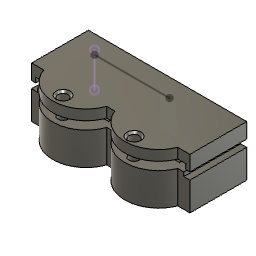
nixie_holder v9 (Autodesk Fusion 360 design; units mm, degrees)
Autodesk Fusion 360 part; units mm, degrees
sketch "Skizze1" plane through (0, 0, 0) normal (0, 1, 0) x (1, 0, 0)
  circle A0 centre (0, 0) radius 7
  circle A1 centre (0, 0) radius 12.5
  line L0 (0, 0) -> (13, 0)
  line L1 (13, 0) -> (13, -2)
  line L2 (13, -2) -> (0, -2)
  line L3 (0, -2) -> (0, 0)
  line L4 (0, 0) -> (-13, 0)
  line L5 (-13, 0) -> (-13, -2)
  line L6 (-13, -2) -> (0, -2)
  line L7 (0, -2) -> (0, 0)
  line L8 (14, -14) -> (-14, -14)
  line L9 (-14, -14) -> (-14, 14)
  line L10 (-14, 14) -> (14, 14)
  line L11 (14, 14) -> (14, -14)
  line L12 (14, -14) -> (-14, 14) construction
  line L13 (-14, -14) -> (14, 14) construction
  line L14 (15.5, 15.5) -> (-15.5, 15.5)
  line L15 (-15.5, 15.5) -> (-15.5, -15.5)
  line L16 (-15.5, -15.5) -> (15.5, -15.5)
  line L17 (15.5, -15.5) -> (15.5, 15.5)
  line L18 (15.5, 15.5) -> (-15.5, -15.5) construction
  line L19 (-15.5, 15.5) -> (15.5, -15.5) construction
  line L20 (-13, -2) -> (-13, -14)
  line L21 (-13, 0) -> (-15.5, 0)
  line L22 (13, -2) -> (14, -2)
  line L23 (13, 0) -> (15.5, 0)
  line L24 (15.5, -2) -> (14, -2)
  line L25 (-13, -2) -> (-15.5, -2)
  line L26 (-15.5, 15.5) -> (15.5, 15.5)
  line L27 (15.5, 15.5) -> (15.5, 14)
  line L28 (15.5, 14) -> (-15.5, 14)
  line L29 (-15.5, 14) -> (-15.5, 15.5)
  dimension "d1" = 14
  dimension "d2" = 25
  dimension "d3" = 28
  dimension "d4" = 31
  dimension "d5" = 31
  constraint coincident A0.centre A1.centre
  constraint horizontal L0
  constraint vertical L1
  constraint horizontal L2
  constraint vertical L3
  constraint horizontal L4
  constraint vertical L5
  constraint horizontal L6
  constraint vertical L7
  constraint perpendicular L8 L9
  constraint parallel L8 L10
  constraint parallel L9 L11
  constraint horizontal L8
  constraint coincident L12 A0.centre
  constraint coincident L13 A0.centre
  constraint perpendicular L14 L15
  constraint parallel L14 L16
  constraint parallel L15 L17
  constraint horizontal L14
  constraint coincident L18 A0.centre
  constraint coincident L19 A0.centre
  constraint perpendicular L6 L20
  constraint midpoint L15 L21.end
  constraint coincident L11 L22.end
  constraint perpendicular L11 L22
  constraint midpoint L17 L23.end
  constraint coincident L17 L24.start
  constraint perpendicular L11 L24
  constraint coincident L15 L25.end
  constraint perpendicular L15 L25
  constraint horizontal L26
  constraint vertical L27
  constraint horizontal L28
  constraint vertical L29
  constraint coincident L17 L27.end
  measures "d1" diameter of A0
  measures "d2" diameter of A1
  measures "d3" distance of L8.end L9.end
  measures "d4" distance of L15.end L16.end
  measures "d5" distance of L14.end L15.end
extrude "Extrusion1" add sketch "Skizze1" along normal blind 12 contours A0 A1 L0 L2 | A0 A1 L0 L4 | A0 A1 L4 L6 | A0 A1 L2 L6 | A1 L0 L1 L2 | A1 L4 L5 L6 | L1 L11 L22 L23 | L5 L9 L21 L25 | L11 L17 L23 L24 | L11 L17 L23 L28 | L9 L15 L21 L28 | L9 L15 L21 L25 | L8 L9 L11 L15 L16 L17 L24 L25 makes body 1
sketch "Skizze2" plane through (0, 12, 0) normal (0, 1, 0) x (-1, 0, 0)
  line L0 (14, 2) -> (12.339, 2)
  arc A0 (12.339, 2) -> (-12.339, 2) centre (0, 0) ccw
  line L1 (-12.339, 2) -> (-14, 2)
  line L2 (-14, 2) -> (-14, 14)
  line L3 (-14, 14) -> (14, 14)
  line L4 (14, 14) -> (14, 2)
  circle A1 centre (0, 0) radius 7
  arc A2 (-12.5, 0) -> (12.5, 0) centre (0, 0) ccw
  line L5 (12.5, 0) -> (14, 0)
  line L6 (14, 0) -> (14, -14)
  line L7 (14, -14) -> (15.5, -14)
  line L8 (15.5, -14) -> (15.5, 15.5)
  line L9 (15.5, 15.5) -> (-15.5, 15.5)
  line L10 (-15.5, 15.5) -> (-15.5, -14)
  line L11 (-15.5, -14) -> (-14, -14)
  line L12 (-14, -14) -> (-14, 0)
  line L13 (-14, 0) -> (-12.5, 0)
  circle A3 centre (0, 0) radius 7
  circle A4 centre (0, 0) radius 8.5
  dimension "d8" = 17
  constraint coincident A0.centre A1.centre
  constraint concentric A3 A4
  measures "d8" diameter of A4
extrude "Extrusion2" cut sketch "Skizze2" against normal blind 15 contours A4 bodies 1
sketch "Skizze3" plane through (0, 12, 0) normal (0, 1, 0) x (-1, 0, 0)
  circle A0 centre (0, 0) radius 8.5
  line L0 (14, 2) -> (12.339, 2)
  arc A1 (12.339, 2) -> (-12.339, 2) centre (0, 0) ccw
  line L1 (-12.339, 2) -> (-14, 2)
  line L2 (-14, 2) -> (-14, 14)
  line L3 (-14, 14) -> (14, 14)
  line L4 (14, 14) -> (14, 2)
  arc A2 (-12.5, 0) -> (12.5, 0) centre (0, 0) ccw
  line L5 (12.5, 0) -> (14, 0)
  line L6 (14, 0) -> (14, -14)
  line L7 (14, -14) -> (15.5, -14)
  line L8 (15.5, -14) -> (15.5, 15.5)
  line L9 (15.5, 15.5) -> (-15.5, 15.5)
  line L10 (-15.5, 15.5) -> (-15.5, -14)
  line L11 (-15.5, -14) -> (-14, -14)
  line L12 (-14, -14) -> (-14, 0)
  line L13 (-14, 0) -> (-12.5, 0)
  line L14 (14, 0) -> (14, 2)
  line L15 (-14, 0) -> (-14, 2)
  line L16 (15.5, -14) -> (14, -14)
  line L17 (14, -14) -> (14, 14)
  line L18 (14, 14) -> (15.5, 14)
  line L19 (15.5, 14) -> (15.5, -14)
  line L20 (-14, -14) -> (-15.5, -14)
  line L21 (-15.5, -14) -> (-15.5, 14)
  line L22 (-15.5, 14) -> (-14, 14)
  line L23 (-14, 14) -> (-14, -14)
  line L24 (15.5, 15.5) -> (-15.5, 15.5)
  line L25 (-15.5, 15.5) -> (-15.5, 14)
  line L26 (-15.5, 14) -> (15.5, 14)
  line L27 (15.5, 14) -> (15.5, 15.5)
  constraint coincident L5.end L6.start
  constraint coincident L0.start L4.end
  constraint coincident L12.end L13.start
  constraint coincident L1.end L2.start
  constraint horizontal L16
  constraint vertical L17
  constraint horizontal L18
  constraint vertical L19
  constraint coincident L3.end L4.start
  constraint coincident L7.end L8.start
  constraint horizontal L20
  constraint vertical L21
  constraint horizontal L22
  constraint vertical L23
  constraint coincident L10 L21.end
  constraint coincident L11.end L12.start
  constraint horizontal L24
  constraint vertical L25
  constraint horizontal L26
  constraint vertical L27
  constraint coincident L8.end L9.start
extrude "Extrusion3" add sketch "Skizze3" along normal blind 5 contours L4 L6 L7 L8 L14 L16 L17 L18 L19 L26 | L2 L10 L11 L12 L15 L20 L21 L22 L23 L26 bodies 1
extrude "Extrusion4" add 1 faces at (-5.1667, 4, 15.5) along direction (0, 0, 1) blind 10 on bodies 1 bodies 1
extrude "Extrusion5" add 1 faces at (-5.1667, 4, 25.5) along direction (0, 0, 1) blind 5 on bodies 1 bodies 1
sketch "Skizze4" plane through (0, 12, 0) normal (0, 1, 0) x (-1, 0, 0)
  line L0 (-15.5, 14) -> (-14, 14)
  line L1 (-14, 14) -> (14, 14)
  line L2 (14, 14) -> (15.5, 14)
  line L3 (15.5, 14) -> (15.5, 30.5)
  line L4 (15.5, 30.5) -> (-15.5, 30.5)
  line L5 (-15.5, 30.5) -> (-15.5, 14)
  circle A0 centre (0, 21) radius 3
  dimension "d17" = 6
  measures "d17" diameter of A0
extrude "Extrusion6" cut sketch "Skizze4" against normal blind 20 contours A0 bodies 1
chamfer "Fase1" distance 2 angle 45 1 edges at (2.797, 12, 22.0848) on bodies 1
chamfer "Fase2" distance 2 angle 45 1 edges at (2.797, 0, 19.9152) on bodies 1
fillet "Abrundung1" radius 6 1 edges at (-15.5, 6, 30.5) on bodies 1
fillet "Abrundung1" radius 6 1 edges at (15.5, 6, 30.5) on bodies 1
sketch "Skizze5" plane through (15.5, 0, 0) normal (1, 0, 0) x (0, 0, -1)
  line L0 (-24.5, 12) -> (-24.5, 0)
  line L1 (-24.5, 0) -> (14, 0)
  line L2 (14, 0) -> (14, 17)
  line L3 (14, 17) -> (-14, 17)
  line L4 (-14, 17) -> (-14, 12)
  line L5 (-14, 12) -> (-24.5, 12)
  line L6 (-14, 17) -> (14, 17)
  line L7 (14, 17) -> (14, 0)
  line L8 (14, 0) -> (-14, 0)
  line L9 (-14, 0) -> (-14, 17)
  constraint horizontal L6
  constraint vertical L7
  constraint horizontal L8
  constraint vertical L9
  constraint coincident L1.end L2.start
  constraint coincident L3.end L4.start
extrude "Extrusion7" add sketch "Skizze5" along normal blind 3 contours L1 L2 L3 L4 L6 L7 L8 L9 bodies 1
sketch "Skizze6" plane through (-15.5, 0, 0) normal (-1, 0, 0) x (0, 0, 1)
  line L0 (24.5, 0) -> (24.5, 12)
  line L1 (24.5, 12) -> (14, 12)
  line L2 (14, 12) -> (14, 17)
  line L3 (14, 17) -> (-14, 17)
  line L4 (-14, 17) -> (-14, 0)
  line L5 (-14, 0) -> (24.5, 0)
  line L6 (14, 17) -> (-14, 17)
  line L7 (-14, 17) -> (-14, 0)
  line L8 (-14, 0) -> (14, 0)
  line L9 (14, 0) -> (14, 17)
  constraint horizontal L6
  constraint vertical L7
  constraint horizontal L8
  constraint vertical L9
  constraint coincident L4.end L5.start
  constraint coincident L2.end L3.start
extrude "Extrusion8" add sketch "Skizze6" along normal blind 3 contours L2 L3 L4 L5 L6 L7 L8 L9 bodies 1
ref_plane "Arbeitsebene1" through (-16.25, 19, 0) normal (0, 1, 0) x (0, 0, 1)
sketch "Skizze7" plane through (-16.25, 19, 0) normal (0, 1, 0) x (1, 0, 0)
  line L0 (-2.25, 14) -> (34.75, 14)
  line L1 (34.75, 14) -> (34.75, -14)
  line L2 (34.75, -14) -> (-2.25, -14)
  line L3 (-2.25, -14) -> (-2.25, 14)
  line L4 (34.75, 14) -> (35.75, 14)
  line L5 (35.75, 14) -> (35.75, -14)
  line L6 (35.75, -14) -> (34.75, -14)
  line L7 (34.75, -14) -> (34.75, 14)
  line L8 (-2.25, 14) -> (-3.25, 14)
  line L9 (-3.25, 14) -> (-3.25, -14)
  line L10 (-3.25, -14) -> (-2.25, -14)
  line L11 (-2.25, -14) -> (-2.25, 14)
  line L12 (-3.25, 14) -> (-5.25, 14)
  line L13 (-5.25, 14) -> (-5.25, -14)
  line L14 (-5.25, -14) -> (-3.25, -14)
  line L15 (-3.25, -14) -> (-3.25, 14)
  line L16 (35.75, 14) -> (37.75, 14)
  line L17 (37.75, 14) -> (37.75, -14)
  line L18 (37.75, -14) -> (35.75, -14)
  line L19 (35.75, -14) -> (35.75, 14)
  point P0 (-2.25, 14)
  point P1 (34.75, -14)
  dimension "d29" = 1
  dimension "d30" = 1
  dimension "d31" = 2
  dimension "d32" = 2
  constraint horizontal L0
  constraint vertical L1
  constraint horizontal L2
  constraint vertical L3
  constraint coincident P1 L1.end
  constraint coincident P0 L0.start
  constraint horizontal L4
  constraint vertical L5
  constraint horizontal L6
  constraint vertical L7
  constraint horizontal L8
  constraint vertical L9
  constraint horizontal L10
  constraint vertical L11
  constraint horizontal L12
  constraint vertical L13
  constraint horizontal L14
  constraint vertical L15
  constraint horizontal L16
  constraint vertical L17
  constraint horizontal L18
  constraint vertical L19
  measures "d29" distance of L0.end L4.end
  measures "d30" distance of P0 L8.end
  measures "d31" distance of L8.end L12.end
  measures "d32" distance of L4.end L16.end
extrude "Extrusion9" add sketch "Skizze7" along normal blind 3 separate body makes body 2
sketch "Skizze8" plane through (18.5, 0, 0) normal (1, 0, 0) x (0, 0, -1)
  line L0 (-14, 0) -> (14, 0)
  line L1 (14, 0) -> (14, 17)
  line L2 (14, 17) -> (-14, 17)
  line L3 (-14, 17) -> (-14, 0)
  line L4 (14, 0) -> (-14, 0)
  line L5 (-14, 0) -> (-14, 15)
  line L6 (-14, 15) -> (14, 15)
  line L7 (14, 15) -> (14, 0)
  constraint horizontal L4
  constraint vertical L5
  constraint horizontal L6
  constraint vertical L7
  constraint coincident L3 L5.end
  constraint coincident L0.end L1.start
extrude "Extrusion10" add sketch "Skizze8" along normal blind 3 contours L0 L1 L3 L4 L5 L6 L7 bodies 1
sketch "Skizze9" plane through (0, 0, -14) normal (0, 0, -1) x (-1, 0, 0)
  line L0 (-21.5, 0) -> (-14, 0)
  line L1 (-14, 0) -> (-14, 17)
  line L2 (-14, 17) -> (-18.5, 17)
  line L3 (-18.5, 17) -> (-18.5, 15)
  line L4 (-18.5, 15) -> (-21.5, 15)
  line L5 (-21.5, 15) -> (-21.5, 0)
  line L6 (18.5, 17) -> (18.5, 0)
  line L7 (-18.5, 15) -> (18.5, 15)
  constraint coincident L3.end L4.start
  constraint coincident L6 L7.end
  constraint perpendicular L3 L7
sketch "Skizze10" plane through (-18.5, 0, 0) normal (-1, 0, 0) x (0, 0, 1)
  line L0 (14, 0) -> (14, 17)
  line L1 (14, 17) -> (-14, 17)
  line L2 (-14, 17) -> (-14, 0)
  line L3 (-14, 0) -> (14, 0)
  line L4 (14, 0) -> (-14, 0)
  line L5 (-14, 0) -> (-14, 15)
  line L6 (-14, 15) -> (14, 15)
  line L7 (14, 15) -> (14, 0)
  point P0 (-14, 15)
  constraint horizontal L4
  constraint vertical L5
  constraint horizontal L6
  constraint vertical L7
  constraint coincident P0 L5.end
  constraint coincident L0.start L3.end
extrude "Extrusion11" add sketch "Skizze10" along normal blind 3 contours L0 L2 L3 L4 L5 L6 L7 bodies 1
sketch "Skizze11" plane through (0, 19, 0) normal (0, -1, 0) x (1, 0, 0)
  line L0 (-21.5, -14) -> (21.5, -14)
  line L1 (21.5, -14) -> (21.5, 14)
  line L2 (21.5, 14) -> (-21.5, 14)
  line L3 (-21.5, 14) -> (-21.5, -14)
  line L4 (-21.5, -14) -> (-19.5, -14)
  line L5 (-19.5, -14) -> (-19.5, 14)
  line L6 (-19.5, 14) -> (-21.5, 14)
  line L7 (-21.5, 14) -> (-21.5, -14)
  line L8 (21.5, 14) -> (19.5, 14)
  line L9 (19.5, 14) -> (19.5, -14)
  line L10 (19.5, -14) -> (21.5, -14)
  line L11 (21.5, -14) -> (21.5, 14)
  dimension "d39" = 2
  dimension "d40" = 2
  constraint horizontal L4
  constraint vertical L5
  constraint horizontal L6
  constraint vertical L7
  constraint coincident L0.start L3.end
  constraint horizontal L8
  constraint vertical L9
  constraint horizontal L10
  constraint vertical L11
  constraint coincident L1.end L2.start
  measures "d39" distance of L0.start L4.end
  measures "d40" distance of L1.end L8.end
extrude "Extrusion12" add sketch "Skizze11" along normal blind 2 contours L0 L2 L3 L4 L5 L6 L7 | L0 L1 L2 L8 L9 L10 L11 bodies 2
extrude "Extrusion13" cut 1 faces at (-20.5, 15, -4.6667) along direction (0, -1, 0) blind 2 on bodies 1 bodies 1
extrude "Extrusion14" cut 1 faces at (-17, 17, 4.6667) along direction (0, -1, 0) blind 2 on bodies 1 bodies 1
extrude "Extrusion15" cut 1 faces at (19.5, 15, 4.6667) along direction (0, -1, 0) blind 2 on bodies 1 bodies 1
extrude "Extrusion16" cut 1 faces at (17, 17, -4.6667) along direction (0, -1, 0) blind 2 on bodies 1 bodies 1
extrude "Extrusion17" add 1 faces at (-11.4814, 12, 19.5849) along direction (0, 1, 0) blind 3 on bodies 1 bodies 1
sketch "Skizze12" plane through (0, 0, 14) normal (0, 0, -1) x (-1, 0, 0)
  line L0 (-14, 0) -> (14, 0)
  line L1 (14, 0) -> (14, 15)
  line L2 (14, 15) -> (-14, 15)
  line L3 (-14, 15) -> (-14, 0)
  line L4 (-14, 15) -> (14, 15)
  line L5 (14, 15) -> (14, 12)
  line L6 (14, 12) -> (-14, 12)
  line L7 (-14, 12) -> (-14, 15)
  point P0 (14, 12)
  constraint horizontal L4
  constraint vertical L5
  constraint horizontal L6
  constraint vertical L7
  constraint coincident P0 L5.end
  constraint coincident L2.end L3.start
extrude "Extrusion18" add sketch "Skizze12" along normal blind 3 contours L1 L2 L3 L4 L5 L6 L7 bodies 1
chamfer "Fase3" distance 3 angle 45 1 edges at (0, 12, 14) on bodies 1
extrude "Extrusion19" add 1 faces at (-14, 9, -9.3333) along direction (1, 0, 0) blind 0.5 on bodies 1 bodies 1
extrude "Extrusion20" add 1 faces at (14, 9, -9.3333) along direction (-1, 0, 0) blind 0.5 on bodies 1 bodies 1
copy_body "Körper kopieren/einfügen1" bodies 1 makes body 3
move_body "Verschieben1" bodies 3 to x (1, 0, 0) y (0, 1, 0) z (0, 0, 1) at (35, 0, 0)
combine "Kombinieren1" operation add target body 1 tool bodies 3
sketch "Skizze13" plane through (0, 15, 0) normal (0, 1, 0) x (-1, 0, 0)
  circle A0 centre (-35, 21) radius 5
  line L0 (-21.5, -14) -> (-13.5, -14)
  line L1 (-13.5, -14) -> (-13.5, 11)
  line L2 (-13.5, 11) -> (13.5, 11)
  line L3 (13.5, 11) -> (13.5, -14)
  line L4 (13.5, -14) -> (18.5, -14)
  line L5 (18.5, -14) -> (18.5, 14)
  line L6 (18.5, 14) -> (15.5, 14)
  line L7 (15.5, 14) -> (15.5, 24.5)
  arc A1 (15.5, 24.5) -> (9.5, 30.5) centre (9.5, 24.5) ccw
  line L8 (9.5, 30.5) -> (-9.5, 30.5)
  arc A2 (-9.5, 30.5) -> (-15.5, 24.5) centre (-9.5, 24.5) ccw
  line L9 (-15.5, 24.5) -> (-15.5, 14)
  line L10 (-15.5, 14) -> (-19.5, 14)
  line L11 (-19.5, 14) -> (-19.5, 24.5)
  arc A3 (-19.5, 24.5) -> (-25.5, 30.5) centre (-25.5, 24.5) ccw
  line L12 (-25.5, 30.5) -> (-44.5, 30.5)
  arc A4 (-44.5, 30.5) -> (-50.5, 24.5) centre (-44.5, 24.5) ccw
  line L13 (-50.5, 24.5) -> (-50.5, 14)
  line L14 (-50.5, 14) -> (-53.5, 14)
  line L15 (-53.5, 14) -> (-53.5, -14)
  line L16 (-53.5, -14) -> (-48.5, -14)
  line L17 (-48.5, -14) -> (-48.5, 11)
  line L18 (-48.5, 11) -> (-21.5, 11)
  line L19 (-21.5, 11) -> (-21.5, -14)
  circle A5 centre (0, 21) radius 5
  circle A6 centre (0, 21) radius 5
  circle A7 centre (-35, 21) radius 5
  constraint concentric A5 A6
  constraint concentric A0 A7
extrude "Extrusion21" add sketch "Skizze13" against normal blind 15 contours A0 A7 | A5 A6 bodies 1
sketch "Skizze14" plane through (0, 15, 0) normal (0, 1, 0) x (-1, 0, 0)
  line L0 (-21.5, -14) -> (-13.5, -14)
  line L1 (-13.5, -14) -> (-13.5, 11)
  line L2 (-13.5, 11) -> (13.5, 11)
  line L3 (13.5, 11) -> (13.5, -14)
  line L4 (13.5, -14) -> (18.5, -14)
  line L5 (18.5, -14) -> (18.5, 14)
  line L6 (18.5, 14) -> (15.5, 14)
  line L7 (15.5, 14) -> (15.5, 24.5)
  arc A0 (15.5, 24.5) -> (9.5, 30.5) centre (9.5, 24.5) ccw
  line L8 (9.5, 30.5) -> (-9.5, 30.5)
  arc A1 (-9.5, 30.5) -> (-15.5, 24.5) centre (-9.5, 24.5) ccw
  line L9 (-15.5, 24.5) -> (-15.5, 14)
  line L10 (-15.5, 14) -> (-19.5, 14)
  line L11 (-19.5, 14) -> (-19.5, 24.5)
  arc A2 (-19.5, 24.5) -> (-25.5, 30.5) centre (-25.5, 24.5) ccw
  line L12 (-25.5, 30.5) -> (-44.5, 30.5)
  arc A3 (-44.5, 30.5) -> (-50.5, 24.5) centre (-44.5, 24.5) ccw
  line L13 (-50.5, 24.5) -> (-50.5, 14)
  line L14 (-50.5, 14) -> (-53.5, 14)
  line L15 (-53.5, 14) -> (-53.5, -14)
  line L16 (-53.5, -14) -> (-48.5, -14)
  line L17 (-48.5, -14) -> (-48.5, 11)
  line L18 (-48.5, 11) -> (-21.5, 11)
  line L19 (-21.5, 11) -> (-21.5, -14)
  circle A4 centre (0, 20) radius 2.5
  circle A5 centre (-35, 20) radius 2.5
  dimension "d62" = 5
  dimension "d63" = 5
  measures "d62" diameter of A4
  measures "d63" diameter of A5
extrude "Extrusion22" cut sketch "Skizze14" against normal blind 15 contours A4 | A5 bodies 1
ref_plane "Arbeitsebene2" through (0, 7.5, 31.5) normal (0, 0, 1) x (1, 0, 0)
sketch "Skizze15" plane through (0, 7.5, 31.5) normal (0, 0, 1) x (1, 0, 0)
  line L0 (-25, 15) -> (60, 15)
  line L1 (60, 15) -> (60, -10)
  line L2 (60, -10) -> (-25, -10)
  line L3 (-25, -10) -> (-25, 15)
  constraint horizontal L0
  constraint vertical L1
  constraint horizontal L2
  constraint vertical L3
extrude "Extrusion23" cut sketch "Skizze15" against normal blind 5 bodies 1
sketch "Skizze16" plane through (0, 15, 0) normal (0, 1, 0) x (-1, 0, 0)
  line L0 (-19.8431, 26.5) -> (-50.1569, 26.5)
  arc A0 (-50.1569, 26.5) -> (-50.5, 24.5) centre (-44.5, 24.5) ccw
  line L1 (-50.5, 24.5) -> (-50.5, 14)
  line L2 (-50.5, 14) -> (-53.5, 14)
  line L3 (-53.5, 14) -> (-53.5, -14)
  line L4 (-53.5, -14) -> (-48.5, -14)
  line L5 (-48.5, -14) -> (-48.5, 11)
  line L6 (-48.5, 11) -> (-21.5, 11)
  line L7 (-21.5, 11) -> (-21.5, -14)
  line L8 (-21.5, -14) -> (-13.5, -14)
  line L9 (-13.5, -14) -> (-13.5, 11)
  line L10 (-13.5, 11) -> (13.5, 11)
  line L11 (13.5, 11) -> (13.5, -14)
  line L12 (13.5, -14) -> (18.5, -14)
  line L13 (18.5, -14) -> (18.5, 14)
  line L14 (18.5, 14) -> (15.5, 14)
  line L15 (15.5, 14) -> (15.5, 24.5)
  arc A1 (15.5, 24.5) -> (15.1569, 26.5) centre (9.5, 24.5) ccw
  line L16 (15.1569, 26.5) -> (-15.1569, 26.5)
  arc A2 (-15.1569, 26.5) -> (-15.5, 24.5) centre (-9.5, 24.5) ccw
  line L17 (-15.5, 24.5) -> (-15.5, 14)
  line L18 (-15.5, 14) -> (-19.5, 14)
  line L19 (-19.5, 14) -> (-19.5, 24.5)
  arc A3 (-19.5, 24.5) -> (-19.8431, 26.5) centre (-25.5, 24.5) ccw
  circle A4 centre (0, 20) radius 2.5
  circle A5 centre (-35, 20) radius 2.5
  arc A6 (15.5, 14) -> (-15.5, 14) centre (0, 8.5795) ccw
  arc A7 (-19.5, 14) -> (-50.5, 14) centre (-35, 7.8095) ccw
  line L20 (-50.5, 14) -> (15.5, 14)
  line L21 (15.5, 14) -> (15.5, 29.3013)
  line L22 (15.5, 29.3013) -> (-50.5, 29.3013)
  line L23 (-50.5, 29.3013) -> (-50.5, 14)
  constraint coincident L17.end L18.start
  constraint coincident L14.end L15.start
  constraint coincident L1.end L2.start
  constraint coincident L18.end L19.start
  constraint horizontal L20
  constraint vertical L21
  constraint horizontal L22
  constraint vertical L23
extrude "Extrusion24" cut sketch "Skizze16" against normal blind 15 contours L0 A0 L1 L19 A3 A7 L23 | L15 A1 L16 A2 L17 A6 L21 bodies 1
extrude "Extrusion25" cut 1 faces at (20.1667, 17, 4.6667) along direction (0, 1, 0) blind 2 on bodies 2 bodies 2
extrude "Extrusion26" add 1 faces at (21.5, 20, -4.6667) along direction (1, 0, 0) blind 35 on bodies 2 bodies 2
sketch "Skizze17" plane through (0, 22, 0) normal (0, 1, 0) x (-1, 0, 0)
  line L0 (-56.5, -14) -> (21.5, -14)
  line L1 (21.5, -14) -> (21.5, 14)
  line L2 (21.5, 14) -> (-56.5, 14)
  line L3 (-56.5, 14) -> (-56.5, -14)
  arc A0 (15.5, 14) -> (-15.5, 14) centre (0, 8.5795) ccw
  arc A1 (-19.5, 14) -> (-50.5, 14) centre (-35, 7.8095) ccw
  point P0 (15.5, 14)
  point P1 (-15.5, 14)
  point P2 (-19.5, 14)
  point P3 (-50.5, 14)
  constraint coincident P1 A0.end
  constraint coincident P0 A0.start
  constraint coincident P3 A1.end
  constraint coincident P2 A1.start
extrude "Extrusion27" add sketch "Skizze17" against normal blind 3 contours L2 A1 | L2 A0 bodies 2
sketch "Skizze18" plane through (0, 22, 0) normal (0, 1, 0) x (-1, 0, 0)
  line L0 (-56.5, -14) -> (21.5, -14)
  line L1 (21.5, -14) -> (21.5, 14)
  line L2 (21.5, 14) -> (15.5, 14)
  arc A0 (15.5, 14) -> (-15.5, 14) centre (0, 8.5795) ccw
  line L3 (-15.5, 14) -> (-19.5, 14)
  arc A1 (-19.5, 14) -> (-50.5, 14) centre (-35, 7.8095) ccw
  line L4 (-50.5, 14) -> (-56.5, 14)
  line L5 (-56.5, 14) -> (-56.5, -14)
  circle A2 centre (0, 20) radius 2.5
  circle A3 centre (-35, 20) radius 2.5
  dimension "d77" = 5
  dimension "d78" = 5
  measures "d77" diameter of A2
  measures "d78" diameter of A3
extrude "Extrusion28" cut sketch "Skizze18" against normal blind 5 contours A2 | A3 bodies 2
extrude "Extrusion29" add 1 faces at (53.8333, 0, 0) along direction (0, -1, 0) blind 1 on bodies 1 bodies 1
sketch "Skizze19" plane through (0, 19, 0) normal (0, -1, 0) x (1, 0, 0)
  circle A0 centre (35, 20) radius 2.5
  circle A1 centre (0, 20) radius 2.5
  line L0 (-15.5, 14) -> (-19.5, 14)
  line L1 (-19.5, 14) -> (-19.5, -14)
  line L2 (-19.5, -14) -> (56.5, -14)
  line L3 (56.5, -14) -> (56.5, 14)
  line L4 (56.5, 14) -> (50.5, 14)
  arc A2 (50.5, 14) -> (19.5, 14) centre (35, 7.8095) ccw
  line L5 (19.5, 14) -> (15.5, 14)
  arc A3 (15.5, 14) -> (-15.5, 14) centre (0, 8.5795) ccw
  line L6 (56.5, 14) -> (53.5, 14)
  line L7 (53.5, 14) -> (53.5, -14)
  line L8 (53.5, -14) -> (56.5, -14)
  line L9 (56.5, -14) -> (56.5, 14)
  point P0 (53.5, -14)
  constraint horizontal L6
  constraint vertical L7
  constraint horizontal L8
  constraint vertical L9
  constraint coincident P0 L7.end
  constraint coincident L3.end L4.start
extrude "Extrusion30" add sketch "Skizze19" along normal blind 3 contours L2 L3 L4 L6 L7 L8 L9 bodies 2
extrude "Extrusion31" cut 1 faces at (53.5, 18, 4.6667) along direction (1, 0, 0) blind 1 on bodies 2 bodies 2
extrude "Extrusion32" cut 1 faces at (55.1667, 16, 4.6667) along direction (0, 1, 0) blind 1 on bodies 2 bodies 2
extrude "Extrusion33" add 1 faces at (17.8333, 22, -4.6667) along direction (0, 1, 0) blind 2 on bodies 2 bodies 2
chamfer "Fase4" distance 1 angle 45 1 edges at (2.3308, 24, 20.904) on bodies 2
chamfer "Fase5" distance 1 angle 45 1 edges at (37.3308, 24, 20.904) on bodies 2
sketch "Skizze20" plane through (0, -1, 0) normal (0, -1, 0) x (1, 0, 0)
  circle A0 centre (0, 20) radius 2.5
  circle A1 centre (35, 20) radius 2.5
  arc A2 (15.5, 14) -> (-15.5, 14) centre (0, 8.5795) ccw
  line L0 (-15.5, 14) -> (-21.5, 14)
  line L1 (-21.5, 14) -> (-21.5, -14)
  line L2 (-21.5, -14) -> (-13.5, -14)
  line L3 (-13.5, -14) -> (-13.5, 0)
  line L4 (-13.5, 0) -> (-12.5, 0)
  arc A3 (-12.5, 0) -> (12.5, 0) centre (0, 0) ccw
  line L5 (12.5, 0) -> (13.5, 0)
  line L6 (13.5, 0) -> (13.5, -14)
  line L7 (13.5, -14) -> (21.5, -14)
  line L8 (21.5, -14) -> (21.5, 0)
  line L9 (21.5, 0) -> (22.5, 0)
  arc A4 (22.5, 0) -> (47.5, 0) centre (35, 0) ccw
  line L10 (47.5, 0) -> (48.5, 0)
  line L11 (48.5, 0) -> (48.5, -14)
  line L12 (48.5, -14) -> (56.5, -14)
  line L13 (56.5, -14) -> (56.5, 14)
  line L14 (56.5, 14) -> (50.5, 14)
  arc A5 (50.5, 14) -> (19.5, 14) centre (35, 7.8095) ccw
  line L15 (19.5, 14) -> (15.5, 14)
  circle A6 centre (35, 0) radius 8.5
  line L16 (21.5, 14) -> (48.5, 14)
  line L17 (48.5, 14) -> (48.5, 2)
  line L18 (48.5, 2) -> (47.339, 2)
  arc A7 (47.339, 2) -> (22.661, 2) centre (35, 0) ccw
  line L19 (22.661, 2) -> (21.5, 2)
  line L20 (21.5, 2) -> (21.5, 14)
  line L21 (13.5, 14) -> (13.5, 2)
  line L22 (13.5, 2) -> (12.339, 2)
  arc A8 (12.339, 2) -> (-12.339, 2) centre (0, 0) ccw
  line L23 (-12.339, 2) -> (-13.5, 2)
  line L24 (-13.5, 2) -> (-13.5, 14)
  line L25 (-13.5, 14) -> (13.5, 14)
  circle A9 centre (0, 0) radius 8.5
  circle A10 centre (0, 20) radius 2
  circle A11 centre (35, 20) radius 2
  dimension "d93" = 4
  dimension "d94" = 4
  constraint concentric A0 A10
  constraint concentric A1 A11
  measures "d93" diameter of A10
  measures "d94" diameter of A11
extrude "Extrusion34" add sketch "Skizze20" against normal blind 10 contours A0 | A1 bodies 1
extrude "Extrusion35" add 2 faces at (21.5, 8.3333, -9.3333) (21.5, 13.6667, -5.6667) along direction (1, 0, 0) blind 0.2 on bodies 1 bodies 1
extrude "Extrusion36" add 1 faces at (-13.5, 8.6667, -9.3333) along direction (1, 0, 0) blind 0.2 on bodies 1 bodies 1
extrude "Extrusion37" cut 2 faces at (55.1667, 17, 4.6667) (-20.1667, 17, -4.6667) along direction (0, 1, 0) blind 1 on bodies 2 bodies 2
extrude "Extrusion38" add 2 faces at (55.1667, 18, 4.6667) (-20.1667, 18, -4.6667) along direction (0, -1, 0) blind 2 on bodies 2 bodies 2
sketch "Skizze21" plane through (0, -1, 0) normal (0, -1, 0) x (1, 0, 0)
  circle A0 centre (35, 20) radius 2
  circle A1 centre (0, 20) radius 2
  arc A2 (15.5, 14) -> (-15.5, 14) centre (0, 8.5795) ccw
  line L0 (-15.5, 14) -> (-21.5, 14)
  line L1 (-21.5, 14) -> (-21.5, -14)
  line L2 (-21.5, -14) -> (-13.3, -14)
  line L3 (-13.3, -14) -> (-13.3, 0)
  line L4 (-13.3, 0) -> (-12.5, 0)
  arc A3 (-12.5, 0) -> (12.5, 0) centre (0, 0) ccw
  line L5 (12.5, 0) -> (13.5, 0)
  line L6 (13.5, 0) -> (13.5, -14)
  line L7 (13.5, -14) -> (21.7, -14)
  line L8 (21.7, -14) -> (21.7, 0)
  line L9 (21.7, 0) -> (22.5, 0)
  arc A4 (22.5, 0) -> (47.5, 0) centre (35, 0) ccw
  line L10 (47.5, 0) -> (48.5, 0)
  line L11 (48.5, 0) -> (48.5, -14)
  line L12 (48.5, -14) -> (56.5, -14)
  line L13 (56.5, -14) -> (56.5, 14)
  line L14 (56.5, 14) -> (50.5, 14)
  arc A5 (50.5, 14) -> (19.5, 14) centre (35, 7.8095) ccw
  line L15 (19.5, 14) -> (15.5, 14)
  circle A6 centre (35, 0) radius 8.5
  line L16 (21.7, 14) -> (48.5, 14)
  line L17 (48.5, 14) -> (48.5, 2)
  line L18 (48.5, 2) -> (47.339, 2)
  arc A7 (47.339, 2) -> (22.661, 2) centre (35, 0) ccw
  line L19 (22.661, 2) -> (21.7, 2)
  line L20 (21.7, 2) -> (21.7, 14)
  line L21 (13.5, 14) -> (13.5, 2)
  line L22 (13.5, 2) -> (12.339, 2)
  arc A8 (12.339, 2) -> (-12.339, 2) centre (0, 0) ccw
  line L23 (-12.339, 2) -> (-13.3, 2)
  line L24 (-13.3, 2) -> (-13.3, 14)
  line L25 (-13.3, 14) -> (13.5, 14)
  circle A9 centre (0, 0) radius 8.5
  circle A10 centre (0, 0) radius 10.5
  circle A11 centre (35, 0) radius 10.5
  dimension "d105" = 21
  dimension "d106" = 21
  constraint coincident A3.centre A8.centre
  constraint concentric A4 A11
  measures "d105" diameter of A10
  measures "d106" diameter of A11
extrude "Extrusion39" cut sketch "Skizze21" against normal blind 16 contours A10 | A11 bodies 1
sketch "Skizze22" plane through (0, -1, 0) normal (0, -1, 0) x (1, 0, 0)
  circle A0 centre (0, 0) radius 10.5
  circle A1 centre (35, 0) radius 10.5
  circle A2 centre (35, 20) radius 2
  circle A3 centre (0, 20) radius 2
  arc A4 (15.5, 14) -> (-15.5, 14) centre (0, 8.5795) ccw
  line L0 (-15.5, 14) -> (-21.5, 14)
  line L1 (-21.5, 14) -> (-21.5, -14)
  line L2 (-21.5, -14) -> (-13.3, -14)
  line L3 (-13.3, -14) -> (-13.3, 0)
  line L4 (-13.3, 0) -> (-12.5, 0)
  arc A5 (-12.5, 0) -> (12.5, 0) centre (0, 0) ccw
  line L5 (12.5, 0) -> (13.5, 0)
  line L6 (13.5, 0) -> (13.5, -14)
  line L7 (13.5, -14) -> (21.7, -14)
  line L8 (21.7, -14) -> (21.7, 0)
  line L9 (21.7, 0) -> (22.5, 0)
  arc A6 (22.5, 0) -> (47.5, 0) centre (35, 0) ccw
  line L10 (47.5, 0) -> (48.5, 0)
  line L11 (48.5, 0) -> (48.5, -14)
  line L12 (48.5, -14) -> (56.5, -14)
  line L13 (56.5, -14) -> (56.5, 14)
  line L14 (56.5, 14) -> (50.5, 14)
  arc A7 (50.5, 14) -> (19.5, 14) centre (35, 7.8095) ccw
  line L15 (19.5, 14) -> (15.5, 14)
  line L16 (21.7, 14) -> (48.5, 14)
  line L17 (48.5, 14) -> (48.5, 2)
  line L18 (48.5, 2) -> (47.339, 2)
  arc A8 (47.339, 2) -> (22.661, 2) centre (35, 0) ccw
  line L19 (22.661, 2) -> (21.7, 2)
  line L20 (21.7, 2) -> (21.7, 14)
  line L21 (13.5, 14) -> (13.5, 2)
  line L22 (13.5, 2) -> (12.339, 2)
  arc A9 (12.339, 2) -> (-12.339, 2) centre (0, 0) ccw
  line L23 (-12.339, 2) -> (-13.3, 2)
  line L24 (-13.3, 2) -> (-13.3, 14)
  line L25 (-13.3, 14) -> (13.5, 14)
  circle A10 centre (0, 0) radius 13.5
  circle A11 centre (35, 0) radius 13.5
  dimension "d109" = 27
  dimension "d110" = 27
  constraint concentric A0 A10
  constraint concentric A1 A11
  measures "d109" diameter of A10
  measures "d110" diameter of A11
extrude "Extrusion40" add sketch "Skizze22" against normal blind 13 contours L3 L4 A5 L5 A10 | L22 A9 L23 L24 A10 | L8 L9 A6 L10 A11 | L18 A8 L19 L20 A11 bodies 1
extrude "Extrusion41" cut 2 faces at (-20.1667, 16, -4.6667) (55.1667, 16, 4.6667) along direction (0, 1, 0) blind 0.5 on bodies 2 bodies 2
